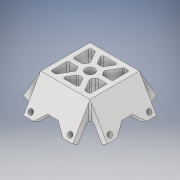
# Autodesk Inventor part: 4-Tool_Upper
Saved by Autodesk Inventor 2019 (Build 230136000, 136)
## iProperties
Created: 2021-01-31
Part Number: 4-Tool_Upper
Material: ABS Plastic
Document SubType Name: Modeling
Designer: zhanb
Density: 1.06 g/cm^3
Appearance: Smooth - White
Author: zhanb
Autodesk Inventor part; units mm, degrees
ref_plane "XZ Plane" through (0, 0, 0) normal (0, 1, 0) x (-1, 0, 0)
ref_plane "XY Plane" through (0, 0, 0) normal (0, 0, 1) x (1, 0, 0)
sketch "Sketch2" plane through (0, 0, 0) normal (1, 0, 0) x (0, 1, 0)
  line L0 (-38.1, 25.4) -> (38.1, 25.4) construction
  line L1 (38.1, 25.4) -> (38.1, -25.4) construction
  line L2 (38.1, -25.4) -> (-38.1, -25.4) construction
  line L3 (-38.1, -25.4) -> (-38.1, 25.4) construction
  line L4 (-38.1, 25.4) -> (38.1, -25.4) construction
  line L5 (38.1, 25.4) -> (-38.1, -25.4) construction
  line L6 (38.1, 25.4) -> (-60.8867, 82.55) construction
  line L7 (-60.8867, 82.55) -> (-67.2367, 71.5515) construction
  line L8 (-67.2367, 71.5515) -> (19.05, 21.7338) construction
  line L9 (38.1, 0) -> (82.0941, 0) construction
  line L10 (82.0941, 0) -> (38.1, 25.4) construction
  line L11 (38.1, 25.4) -> (7.3041, 43.18)
  line L12 (7.3041, 43.18) -> (4.1291, 37.6807)
  line L13 (0.9541, 32.1815) -> (0.9541, 0) construction
  line L14 (0.9541, 0) -> (19.05, 0) construction
  line L15 (38.1, 25.4) -> (38.1, 0)
  line L16 (0.9541, 32.1815) -> (19.05, 21.7338) construction
  line L17 (19.05, 21.7338) -> (19.05, 0)
  line L18 (19.05, 0) -> (38.1, 0)
  line L19 (4.1291, 37.6807) -> (19.05, 29.0662)
  line L20 (19.05, 29.0662) -> (19.05, 21.7338)
  line L21 (4.1291, 37.6807) -> (0.9541, 32.1815) construction
  point P0 (0, 0)
  dimension "d2" = 76.2
  dimension "d3" = 50.8
  dimension "d4" = 12.7
  dimension "d5" = 30
  dimension "d6" = 114.3
  dimension "d7" = 35.56
  dimension "d32" = 6.35
  dimension "d51" = 19.05
  constraints: 44 end point, 11 perpendicular, 3 collinear, 3 midpoint, 3 parallel, 2 horizontal, 2 point on line
  measures "d2" distance of L1.end L2.end
  measures "d3" distance of L0.end L1.end
  measures "d4" distance of L6.end L7.end
  measures "d5" angle of L9 L10
  measures "d6" distance of L0.end L6.end
  measures "d7" distance of L0.end L11.end
  measures "d32" distance between parallel lines of L11 L19
  measures "d51" distance between parallel lines of L17 L15
extrude "Extrusion1" add sketch "Sketch2" along normal mid plane 50.8
pattern_circular "Circular Pattern1" count 4 over 360 about axis through (0, -10, 0) along (0, 1, 0) of "Extrusion1"
sketch "Sketch5" plane through (-25.4, 38.1, -25.4) normal (-0.8660254, 0.5, 0) x (0, 0, 1)
  circle A0 centre (5.08, -30.48) radius 2.5527
  circle A1 centre (45.72, -30.48) radius 2.5527
  line L0 (5.08, -30.48) -> (45.72, -30.48) construction
  line L1 (50.8, 0) -> (0, 0) construction
  point P0 (25.4, -30.48)
  point P1 (25.4, 0)
  dimension "d20" = 40.64
  dimension "d21" = 5.1054
  dimension "d22" = 5.1054
  dimension "d24" = 30.48
  constraints: 2 centre point, 2 coincident, 2 end point, 2 midpoint, 1 horizontal, 1 horizontal alignment, 1 vertical alignment
  measures "d20" distance of point (45.72, -30.48) point (5.08, -30.48)
  measures "d21" diameter of A0
  measures "d22" diameter of A1
  measures "d24" distance from line of L1 point (25.4, -30.48)
hole "Hole1" at (-40.64, 11.7035, -20.32) at (-40.64, 11.7035, 20.32) direction (0.8660254, -0.5, 0) diameter 5.1562 end through all
sketch "Sketch6" plane through (0, 0, 0) normal (0, 0, 1) x (1, 0, 0)
  line L0 (-32.7323, 12.7) -> (-25.1123, 12.7)
  line L1 (-25.1123, 12.7) -> (-21.4462, 19.05)
  line L2 (25.4, 19.05) -> (-25.4, 19.05) construction
  line L3 (-29.0662, 19.05) -> (-32.7323, 12.7)
  line L4 (-37.6807, 4.1291) -> (-29.0662, 19.05) construction
  line L5 (-29.0662, 19.05) -> (-21.4462, 19.05)
  point P0 (0, 0)
  dimension "d34" = 6.35
  dimension "d35" = 7.62
  constraints: 8 end point, 2 collinear, 1 horizontal, 1 parallel, 1 point on line
  measures "d34" distance between parallel lines of L5 L0
  measures "d35" distance of L3.start L1.end
extrude "Extrusion3" add sketch "Sketch6" along normal mid plane 5.08
sketch "Sketch7" plane through (-43.18, 7.3041, -25.4) normal (-0.8660254, 0.5, 0) x (0, 0, 1)
  line L0 (22.86, 9.8968) -> (27.94, 9.8968) construction
  line L1 (10.16, 0) -> (20.0568, 9.8968)
  line L2 (20.0568, 9.8968) -> (30.7432, 9.8968)
  line L3 (30.7432, 9.8968) -> (40.64, 0)
  line L4 (40.64, 0) -> (10.16, 0)
  line L5 (0, 0) -> (50.8, 0) construction
  point P0 (25.4, 15.2644)
  point P1 (25.4, 9.8968)
  point P2 (25.4, 0)
  dimension "d38" = 45
  dimension "d39" = 10.16
  constraints: 8 end point, 4 midpoint, 3 collinear, 1 horizontal
  measures "d38" angle of L4 L1
  measures "d39" distance of L5.start L1.start
extrude "Extrusion4" cut sketch "Sketch7" against normal through all
sketch "Sketch8" plane through (-25.4, 38.1, 25.4) normal (0, 1, 0) x (1, 0, 0)
  line L0 (28.1643, 20.6121) -> (22.6357, 20.6121) construction
  line L1 (22.6357, 20.6121) -> (19.8714, 25.4) construction
  line L2 (19.8714, 25.4) -> (22.6357, 30.1879) construction
  line L3 (22.6357, 30.1879) -> (28.1643, 30.1879) construction
  line L4 (28.1643, 30.1879) -> (30.9286, 25.4) construction
  line L5 (30.9286, 25.4) -> (28.1643, 20.6121) construction
  line L6 (45.72, 45.72) -> (5.08, 45.72) construction
  line L7 (5.08, 45.72) -> (5.08, 5.08) construction
  line L8 (5.08, 5.08) -> (45.72, 5.08) construction
  line L9 (45.72, 5.08) -> (45.72, 45.72) construction
  line L10 (45.72, 45.72) -> (5.08, 5.08) construction
  line L11 (5.08, 45.72) -> (45.72, 5.08) construction
  line L12 (35.328, 22.86) -> (45.72, 22.86)
  line L13 (45.72, 22.86) -> (45.72, 5.08)
  line L14 (45.72, 5.08) -> (40.0647, 5.08)
  line L15 (40.0647, 5.08) -> (32.5637, 18.0721)
  line L16 (32.5637, 18.0721) -> (35.328, 22.86)
  line L17 (28.1643, 15.5321) -> (22.6357, 15.5321)
  line L18 (22.6357, 15.5321) -> (16.6012, 5.08)
  line L19 (34.1988, 5.08) -> (28.1643, 15.5321)
  line L20 (28.1643, 20.6121) -> (37.1318, 5.08) construction
  line L21 (10.7353, 5.08) -> (18.2363, 18.0721)
  line L22 (18.2363, 18.0721) -> (15.472, 22.86)
  line L23 (15.472, 22.86) -> (5.08, 22.86)
  line L24 (5.08, 22.86) -> (5.08, 5.08)
  line L25 (10.7353, 5.08) -> (5.08, 5.08)
  line L26 (45.72, 27.94) -> (35.328, 27.94)
  line L27 (35.328, 27.94) -> (32.5637, 32.7279)
  line L28 (32.5637, 32.7279) -> (40.0647, 45.72)
  line L29 (40.0647, 45.72) -> (45.72, 45.72)
  line L30 (45.72, 27.94) -> (45.72, 45.72)
  line L31 (30.9286, 25.4) -> (45.72, 25.4) construction
  line L32 (31.0972, 15.5321) -> (19.7028, 15.5321) construction
  line L33 (19.7028, 15.5321) -> (14.0055, 25.4) construction
  line L34 (14.0055, 25.4) -> (19.7028, 35.2679) construction
  line L35 (19.7028, 35.2679) -> (31.0972, 35.2679) construction
  line L36 (31.0972, 35.2679) -> (36.7945, 25.4) construction
  line L37 (36.7945, 25.4) -> (31.0972, 15.5321) construction
  line L38 (14.0055, 25.4) -> (5.08, 25.4) construction
  line L39 (25.4, 5.08) -> (25.4, 25.4) construction
  line L40 (28.1643, 35.2679) -> (34.1988, 45.72)
  line L41 (16.6012, 45.72) -> (22.6357, 35.2679)
  line L42 (28.1643, 35.2679) -> (22.6357, 35.2679)
  line L43 (15.472, 27.94) -> (5.08, 27.94)
  line L44 (5.08, 27.94) -> (5.08, 45.72)
  line L45 (5.08, 45.72) -> (10.7353, 45.72)
  line L46 (10.7353, 45.72) -> (18.2363, 32.7279)
  line L47 (15.472, 27.94) -> (18.2363, 32.7279)
  line L48 (31.0972, 35.2679) -> (37.1318, 45.72) construction
  line L49 (30.4483, 11.576) -> (34.8477, 14.116) construction
  line L50 (34.1988, 5.08) -> (16.6012, 5.08)
  line L51 (34.1988, 45.72) -> (16.6012, 45.72)
  circle A0 centre (25.4, 25.4) radius 4.7879
  point P0 (25.4, 15.5321)
  point P1 (25.4, 20.6121)
  point P2 (32.648, 12.846)
  point P3 (25.4, 30.1879)
  dimension "d42" = 9.5758
  dimension "d46" = 40.64
  dimension "d47" = 40.64
  dimension "d48" = 5.08
  dimension "d49" = 5.08
  dimension "d50" = 5.08
  constraints: 104 end point, 12 point on line, 11 equal length, 10 horizontal, 10 midpoint, 9 perpendicular, 8 parallel, 7 collinear, 3 coincident, 2 vertical alignment, 1 vertical, 33 other
  measures "d42" distance between parallel lines of L3 L0
  measures "d46" distance of L6.end L7.end
  measures "d47" distance of L7.end L8.end
  measures "d48" distance of L49.start L49.end
  measures "d49" distance between parallel lines of L26 L12
  measures "d50" distance between parallel lines of L5 L16
extrude "Extrusion5" cut sketch "Sketch8" against normal through all
fillet "Fillet1" radius 1.5875 28 edges at (-2.7643, 28.575, -9.8679) (2.7643, 28.575, -9.8679) (8.7988, 28.575, -20.32) (-8.7988, 28.575, -20.32) (-20.32, 28.575, 20.32) (-14.6647, 28.575, 20.32) (-7.1637, 28.575, 7.3279) (-9.928, 28.575, 2.54) (-20.32, 28.575, 2.54) (14.6647, 28.575, 20.32) (20.32, 28.575, 20.32) (20.32, 28.575, 2.54) (9.928, 28.575, 2.54) (7.1637, 28.575, 7.3279) (8.7988, 28.575, 20.32) (2.7643, 28.575, 9.8679) (-2.7643, 28.575, 9.8679) (-8.7988, 28.575, 20.32) (7.1637, 28.575, -7.3279) (9.928, 28.575, -2.54) (20.32, 28.575, -2.54) (20.32, 28.575, -20.32) (14.6647, 28.575, -20.32) (-20.32, 28.575, -20.32) (-20.32, 28.575, -2.54) (-9.928, 28.575, -2.54) (-7.1637, 28.575, -7.3279) (-14.6647, 28.575, -20.32)
pattern_circular "Circular Pattern2" count 4 over 360 about axis through (0, -10, 0) along (0, 1, 0) of "Extrusion3", "Hole1", "Extrusion4"
fillet "Fillet2" radius 1.5875 12 edges at (-25.4, 28.575, -25.4) (-25.4, 28.575, 25.4) (25.4, 28.575, 25.4) (25.4, 28.575, -25.4) (29.0662, 19.05, -13.97) (13.97, 19.05, -29.0662) (-13.97, 19.05, -29.0662) (29.0662, 19.05, 13.97) (13.97, 19.05, 29.0662) (-13.97, 19.05, 29.0662) (-29.0662, 19.05, 13.97) (-29.0662, 19.05, -13.97)
sketch "Sketch9" plane through (-21.4462, 19.05, -2.54) normal (0, -1, 0) x (1, 0, 0)
  circle A0 centre (21.4462, 2.54) radius 6.35
  circle A1 centre (21.4462, 2.54) radius 4.7879 projected
  dimension "d54" = 12.7
  constraints: 1 centre point, 1 coincident
  measures "d54" diameter of A0
extrude "Extrusion6" add sketch "Sketch9" along normal blind 6.35
ref_plane "Work Plane1" through (0, 0, 0) normal (0.7071068, 0, -0.7071068) x (0, 1, 0)
sketch "Sketch11" plane through (0, 0, 0) normal (0.7071068, 0, -0.7071068) x (0, 1, 0)
  line L0 (19.05, -6.35) -> (19.05, 6.35) construction
  line L1 (12.7, 6.35) -> (19.05, 6.35) construction
  line L2 (19.05, 6.35) -> (19.05, -6.35) construction
  line L3 (19.05, -6.35) -> (12.7, -6.35) construction
  line L4 (12.7, -6.35) -> (12.7, 6.35) construction
  line L5 (12.7, 6.35) -> (19.05, -6.35) construction
  line L6 (19.05, 6.35) -> (12.7, -6.35) construction
  line L7 (12.7, 6.35) -> (12.7, -6.35) construction
  circle A0 centre (15.875, 0) radius 0.7938
  point P0 (0, 0)
  dimension "d61" = 1.5875
  constraints: 12 end point, 2 midpoint, 2 parallel, 1 centre point, 1 coincident, 1 horizontal, 1 perpendicular, 1 point on line
  measures "d61" diameter of A0
extrude "Extrusion8" cut sketch "Sketch11" along normal mid plane 15.875
fillet "Fillet3" radius 1.5875 1 edges at (-6.35, 19.05, 0)
equation "\"d47\" = d46"
equation "\"d49\" = d48"
equation "\"d50\" = d48"
body "Solid1"
